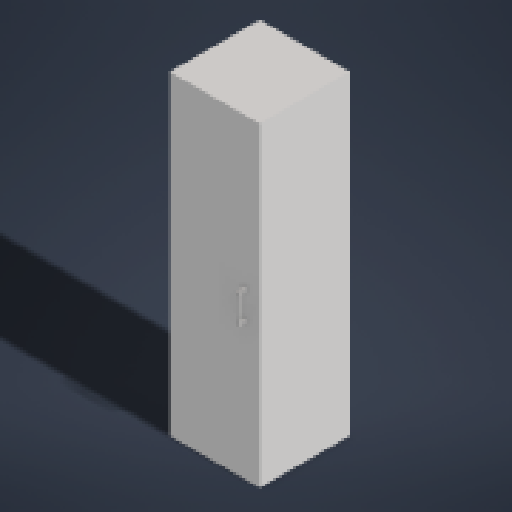
# Autodesk Inventor part: Frigorifero
Saved by Autodesk Inventor 2024.2 (Build 282272000, 272)
## iProperties
Created: 2025-08-13
Part Number: Frigorifero
Material: Generic
Document SubType Name: Modeling
Designer: Luca
Density: 1 g/cm^3
Appearance: Default
Author: Luca
Autodesk Inventor part; units mm, degrees
ref_plane "YZ Plane" through (0, 0, 0) normal (1, 0, 0) x (0, 1, 0)
ref_plane "XZ Plane" through (0, 0, 0) normal (0, 1, 0) x (-1, 0, 0)
sketch "Sketch1" plane through (0, 0, 0) normal (0, 1, 0) x (-1, 0, 0)
  line L0 (300, 600) -> (-300, 600)
  line L1 (-300, 600) -> (-300, 0)
  line L2 (-300, 0) -> (300, 0)
  line L3 (300, 0) -> (300, 600)
  point P0 (0, 0)
  point P1 (0, 0)
  dimension "d0" = 600
  dimension "d1" = 600
  constraints: 8 end point, 2 parallel, 1 coincident, 1 horizontal, 1 midpoint, 1 perpendicular
  measures "d0" distance of L2.end L1.end
  measures "d1" distance of L1.end L0.end
extrude "Extrusion1" add sketch "Sketch1" along normal blind 2100
ref_plane "Work Plane1" through (200, 0, 600) normal (1, 0, 0) x (0, 0, -1)
sketch "Sketch2" plane through (200, 0, 600) normal (1, 0, 0) x (0, 0, -1)
  line L0 (0, 1106.8503) -> (-50, 1106.8503)
  line L1 (-50, 1106.8503) -> (-50, 906.8503)
  line L2 (-50, 906.8503) -> (0, 906.8503)
  line L3 (0, 906.8503) -> (0, 926.8503)
  line L4 (0, 926.8503) -> (-39.8997, 926.8503)
  line L5 (-39.8997, 926.8503) -> (-39.8997, 1086.8503)
  line L6 (-39.8997, 1086.8503) -> (0, 1086.8503)
  line L7 (0, 1086.8503) -> (0, 1106.8503)
  line L8 (0, 0) -> (0, 2100) projected
  point P0 (600, 0)
  dimension "d5" = 20
  dimension "d6" = 200
  dimension "d7" = 50
  constraints: 16 end point, 7 perpendicular, 2 collinear, 1 horizontal, 1 point on line
  measures "d5" distance between parallel lines of L0 L6
  measures "d6" distance of L0.end L1.end
  measures "d7" distance between parallel lines of L8 L1
extrude "Extrusion2" add sketch "Sketch2" along normal mid plane 20 contours L7 L6 L5 L4 L3 L2 L1 L0
equation "\"d8\" = d5"
body "Solid1"
